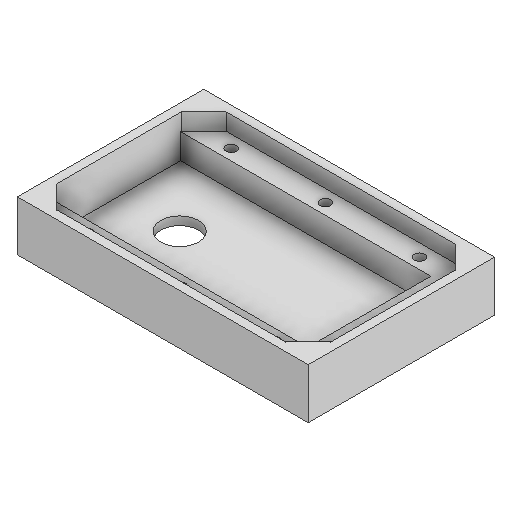
# Autodesk Inventor part: mx-106
Saved by Autodesk Inventor 2025.2 (Build 292293000, 293)
## iProperties
Created: 2025-06-17
Part Number: mx-106
Material: 일반
Document SubType Name: Modeling
Designer: joseph
Density: 1 g/cm^3
Appearance: 기본값
Author: joseph
Autodesk Inventor part; units mm, degrees
ref_plane "YZ Plane" through (0, 0, 0) normal (1, 0, 0) x (0, 1, 0)
ref_plane "XZ Plane" through (0, 0, 0) normal (0, 1, 0) x (-1, 0, 0)
ref_plane "XY Plane" through (0, 0, 0) normal (0, 0, 1) x (1, 0, 0)
sketch "스케치1" plane through (0, 0, 0) normal (0, 1, 0) x (-1, 0, 0)
  line L0 (0, 0) -> (65.45, 0)
  line L1 (65.45, 0) -> (65.45, -40.5)
  line L2 (65.45, -40.5) -> (0, -40.5)
  line L3 (0, -40.5) -> (0, 0)
  line L4 (67.45, -42.5) -> (67.45, 2)
  line L5 (67.45, 2) -> (-2, 2)
  line L6 (-2, 2) -> (-2, -42.5)
  line L7 (-2, -42.5) -> (67.45, -42.5)
  line L8 (65.45, -20.25) -> (0, -20.25) construction
  line L9 (32.725, 0) -> (32.725, -40.5) construction
  line L10 (65.45, -5.4) -> (60.05, 0)
  line L11 (65.45, -35.1) -> (60.05, -40.5)
  line L12 (0, 0) -> (0, -40.5)
  line L13 (0, -5.4) -> (5.4, 0)
  line L14 (0, -35.1) -> (5.4, -40.5)
  dimension "d0" = 65.45
  dimension "d1" = 40.5
  dimension "d2" = 2
  dimension "d3" = 5.4
  dimension "d4" = 5.4
  constraints: 30 end point, 6 symmetric about line, 4 midpoint, 4 parallel, 3 point on line, 2 perpendicular, 1 horizontal, 3 other
  measures "d0" distance of L1.end L2.end
  measures "d1" distance of L0.end L1.end
  measures "d2" distance between parallel lines of L1 L4
  measures "d3" distance of L10.start L0.end
  measures "d4" distance of L10.end L0.end
extrude "돌출1" add sketch "스케치1" along normal blind 10 contours L0 L13 L3 | L0 L1 L10 | L14 L2 L3 | L1 L2 L11 | L7 L6 L5 L4
sketch "스케치2" plane through (0, 0, 0) normal (0, -1, 0) x (1, 0, 0)
  line L0 (-67.45, 2) -> (2, 2) projected
  line L1 (-67.45, -42.5) -> (-67.45, 2) projected
  line L2 (2, -42.5) -> (-67.45, -42.5) projected
  line L3 (2, 2) -> (2, -42.5) projected
  line L4 (0, -5.4) -> (-5.4, 0) projected
  line L5 (0, -35.1) -> (0, -5.4) projected
  line L6 (-60.05, -40.5) -> (-5.4, -40.5) projected
  line L7 (-65.45, -5.4) -> (-65.45, -35.1) projected
  line L8 (-5.4, 0) -> (-60.05, 0) projected
  line L9 (-5.4, -40.5) -> (0, -35.1) projected
  line L10 (-65.45, -35.1) -> (-60.05, -40.5) projected
  line L11 (-60.05, 0) -> (-65.45, -5.4) projected
  point P0 (0, 0)
extrude "돌출2" add sketch "스케치2" along normal blind 2 contours L0 L3 L2 L1 | L5 L9 L6 L10 L7 L11 L8 L4
sketch "스케치3" plane through (0, 0, 0) normal (0, 1, 0) x (1, 0, 0)
  line L0 (0, 35.1) -> (0, 5.4) projected
  line L1 (-5.4, 40.5) -> (0, 35.1) projected
  line L2 (-60.05, 40.5) -> (-5.4, 40.5) projected
  line L3 (-65.45, 35.1) -> (-60.05, 40.5) projected
  line L4 (-65.45, 5.4) -> (-65.45, 35.1) projected
  line L5 (-60.05, 0) -> (-65.45, 5.4) projected
  line L6 (-5.4, 0) -> (-60.05, 0) projected
  line L7 (0, 5.4) -> (-5.4, 0) projected
  line L8 (-65.45, 5.4) -> (-65.45, 35.1) projected
  line L9 (-65.45, 5.55) -> (-5.65, 5.55)
  line L10 (-5.65, 5.55) -> (-5.65, 34.95)
  line L11 (-5.65, 34.95) -> (-65.45, 34.95)
  line L12 (-65.45, 34.95) -> (-65.45, 5.55)
  line L13 (0, 35.1) -> (0, 5.4) projected
  line L14 (-5.4, 40.5) -> (0, 35.1) projected
  line L15 (-60.05, 40.5) -> (-5.4, 40.5) projected
  line L16 (-65.45, 35.1) -> (-60.05, 40.5) projected
  line L17 (-65.45, 5.4) -> (-65.45, 35.1) projected
  line L18 (-60.05, 0) -> (-65.45, 5.4) projected
  line L19 (-5.4, 0) -> (-60.05, 0) projected
  line L20 (0, 5.4) -> (-5.4, 0) projected
  point P0 (0, 0)
  point P1 (-5.65, 20.25)
  point P2 (-65.45, 20.25)
  dimension "d9" = 59.8
  dimension "d10" = 29.4
  constraints: 8 end point, 2 midpoint, 2 parallel, 1 horizontal, 1 horizontal alignment, 1 perpendicular, 1 point on line
  measures "d9" distance of L10.end L11.end
  measures "d10" distance of L9.end L10.end
extrude "돌출3" add sketch "스케치3" along normal blind 6 contours L0 L7 L6 L5 L4 L9 L10 L11 L3 L2 L1
sketch "스케치4" plane through (0, 0, 0) normal (0, 1, 0) x (1, 0, 0)
  line L0 (-5.65, 34.95) -> (-65.45, 34.95) projected
  line L1 (-65.45, 5.55) -> (-65.45, 34.95) projected
  line L2 (-65.45, 5.55) -> (-5.65, 5.55) projected
  line L3 (-5.65, 5.55) -> (-5.65, 34.95) projected
  circle A0 centre (-50.95, 20.25) radius 4.5
  point P0 (0, 0)
  dimension "d14" = 9
  dimension "d17" = 14.5
  constraints: 1 centre point
  measures "d14" diameter of A0
  measures "d17" distance from line of A0.centre L1
extrude "돌출4" cut sketch "스케치4" against normal blind 6 contours A0
sketch "스케치5" plane through (0, 6, 0) normal (0, 1, 0) x (1, 0, 0)
  line L0 (-5.65, 5.55) -> (-65.45, 5.55) projected
  line L1 (-65.45, 5.4) -> (-65.45, 5.55) projected
  line L2 (-60.05, 0) -> (-65.45, 5.4) projected
  line L3 (-5.4, 0) -> (-60.05, 0) projected
  line L4 (0, 5.4) -> (-5.4, 0) projected
  line L5 (0, 35.1) -> (0, 5.4) projected
  line L6 (-5.4, 40.5) -> (0, 35.1) projected
  line L7 (-60.05, 40.5) -> (-5.4, 40.5) projected
  line L8 (-65.45, 35.1) -> (-60.05, 40.5) projected
  line L9 (-65.45, 34.95) -> (-65.45, 35.1) projected
  line L10 (-65.45, 34.95) -> (-5.65, 34.95) projected
  line L11 (-5.65, 34.95) -> (-5.65, 5.55) projected
  line L12 (-10.4708, 2.95) -> (-58.727, 2.95) construction
  circle A0 centre (-55.95, 2.95) radius 1.25
  line L13 (-67.45, 42.5) -> (-67.45, -2) projected
  circle A1 centre (-33.45, 2.95) radius 1.25
  circle A2 centre (-10.95, 2.95) radius 1.25
  line L14 (-65.45, 5.55) -> (-65.45, 34.95) construction
  line L15 (-65.45, 20.25) -> (-5.65, 20.25) construction
  circle A3 centre (-55.95, 37.55) radius 1.25
  circle A4 centre (-33.45, 37.55) radius 1.25
  circle A5 centre (-10.95, 37.55) radius 1.25
  point P0 (0, 0)
  point P1 (-10.4708, 37.55)
  dimension "d18" = 2.5
  dimension "d19" = 11.5
  dimension "d22" = 22.5
  dimension "d27" = 34.6
  constraints: 6 centre point, 4 end point, 4 symmetric about line, 2 horizontal, 2 midpoint, 1 point on line, 7 other
  measures "d18" diameter of A0
  measures "d19" distance from line of L13 A0.centre
  measures "d22" distance of A0.centre A1.centre
  measures "d27" distance of A3.centre A0.centre
extrude "돌출5" cut sketch "스케치5" against normal through all contours A0 | A1 | A2 | A3 | A4 | A5
sketch "스케치6" plane through (-65.45, 0, -34.95) normal (0, 0, 1) x (1, 0, 0)
  point P0 (65.45, 0)
